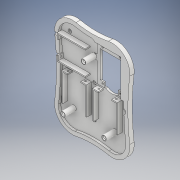
# Autodesk Inventor part: Chwytaka2_o
Saved by Autodesk Inventor 2017 (Build 210142000, 142)
## iProperties
Created: 2014-11-15
Part Number: Chwytaka2_o
Material: SolidWorks Materials|ABS
Document SubType Name: Modeling
Designer: Maciej
Density: 1.02 g/cm^3
Appearance: 255,255,255
Sending System: SolidWorks 2013
Last Author: Raymond Ma
Last Saved: 2015-02-18
Author: Maciej
Autodesk Inventor part; units mm, degrees
note: some values were not read from the file. Chosen so that the rebuilt part matches the saved one: arc direction of "Wyciągnięcie proste15".
ref_plane "YZ Plane" through (0, 0, 0) normal (1, 0, 0) x (0, 1, 0)
ref_plane "XZ Plane" through (0, 0, 0) normal (0, 1, 0) x (-1, 0, 0)
ref_plane "XY Plane" through (0, 0, 0) normal (0, 0, 1) x (1, 0, 0)
sketch "Szkic3" plane through (0, 0, 0) normal (0, 1, 0) x (-1, 0, 0)
  arc A0 (47.3256, 42.282) -> (47.3256, -32.282) centre (345, 5) ccw projected
  arc A1 (47.3256, -32.282) -> (47.3256, -32.282) centre (345, 5) ccw
  arc A2 (20.4082, -57.1046) -> (47.3256, -32.282) centre (25, -35.0782) ccw projected
  arc A3 (20.4082, -57.1046) -> (47.3256, -32.282) centre (25, -35.0782) ccw
  arc A4 (20.4082, -57.1046) -> (-20.4082, -57.1046) centre (0, -155) ccw projected
  arc A5 (20.4082, -57.1046) -> (-20.4082, -57.1046) centre (0, -155) ccw
  arc A6 (-47.3256, -32.282) -> (-20.4082, -57.1046) centre (-25, -35.0782) ccw projected
  arc A7 (-47.3256, -32.282) -> (-47.3256, -32.282) centre (-25, -35.0782) ccw
  arc A8 (-47.3256, -32.282) -> (-47.3256, 42.282) centre (-345, 5) ccw projected
  arc A9 (-47.3256, -32.282) -> (-47.3256, -32.282) centre (-345, 5) ccw
  arc A10 (-20.4082, 67.1046) -> (-47.3256, 42.282) centre (-25, 45.0782) ccw projected
  arc A11 (-20.4082, 67.1046) -> (-47.3256, 42.282) centre (-25, 45.0782) ccw
  arc A12 (-20.4082, 67.1046) -> (20.4082, 67.1046) centre (0, 165) ccw projected
  arc A13 (47.3256, 42.282) -> (20.4082, 67.1046) centre (25, 45.0782) ccw projected
  arc A14 (20.4082, 67.1046) -> (20.4082, 67.1046) centre (0, 165) ccw
  arc A15 (47.3256, 42.282) -> (20.4082, 67.1046) centre (25, 45.0782) ccw
  circle A16 centre (26, -30.3974) radius 1.5 projected
  circle A17 centre (26, -30.3974) radius 1.5
  circle A18 centre (26, -30.3974) radius 3
  circle A19 centre (-26, -30.3974) radius 1.5 projected
  circle A20 centre (-26, -30.3974) radius 1.5
  circle A21 centre (-26, -30.3974) radius 3
  circle A22 centre (-39, 0) radius 2.1526 projected
  circle A23 centre (-39, 0) radius 2.1526
  circle A24 centre (0, 10) radius 2.1526 projected
  circle A25 centre (0, 10) radius 2.1526
  circle A26 centre (31.0104, 51.0886) radius 2.1526 projected
  circle A27 centre (31.0104, 51.0886) radius 2.1526
  circle A28 centre (0, -30.3974) radius 2.1526
  circle A29 centre (0, 40) radius 1.5 projected
  circle A30 centre (0, 40) radius 1.5
  circle A31 centre (0, 40) radius 3
  arc A32 (-27.8847, 10.4357) -> (-15.5153, 10.4357) centre (-21.7, 22.4357) ccw projected
  circle A33 centre (-21.7, 22.4357) radius 13.5
  arc A34 (0, 60) -> (-3.7, 55.3715) centre (1.296, 55.1709) ccw
  arc A35 (-5.5975, 60.1493) -> (21.4286, 62.2098) centre (0, 165) ccw projected
  arc A36 (0, 60) -> (2.4776, 60.0292) centre (0, 165) ccw
  arc A37 (2.4776, 60.0292) -> (21.4286, 62.2098) centre (0, 165) ccw
  arc A38 (42.3644, 42.9034) -> (21.4286, 62.2098) centre (25, 45.0782) ccw projected
  arc A39 (42.3644, 42.9034) -> (40.5404, 23.1486) centre (345, 5) ccw
  arc A40 (21.4286, -52.2098) -> (42.3644, -32.9034) centre (25, -35.0782) ccw projected
  arc A41 (-42.3644, -32.9034) -> (-21.4286, -52.2098) centre (-25, -35.0782) ccw projected
  arc A42 (-42.3644, -32.9034) -> (-40.1293, -3.8798) centre (-345, 5) ccw projected
  arc A43 (-42.3644, -32.9034) -> (-21.4286, -52.2098) centre (-25, -35.0782) ccw
  arc A44 (-42.3644, -32.9034) -> (-40.1293, -3.8798) centre (-345, 5) ccw
  arc A45 (-40.1293, -3.8798) -> (-40.645, -2.9755) centre (-41.1289, -3.8507) ccw projected
  arc A46 (-40.5469, 3.0277) -> (-40.645, -2.9755) centre (-39, 0) ccw projected
  arc A47 (-40.645, -2.9755) -> (-40.645, -2.9755) centre (-39, 0) ccw
  arc A48 (-40.5469, 3.0277) -> (-40.0019, 3.9146) centre (-41.0019, 3.9182) ccw projected
  arc A49 (21.4286, -52.2098) -> (-21.4286, -52.2098) centre (0, -155) ccw
  line L0 (-7.45, 51.4857) -> (-7.45, 17.3857)
  line L1 (-7.45, 11.1857) -> (-35.95, 11.1857)
  line L2 (-3.7, 55.3715) -> (-3.7, 44) projected
  line L3 (-3.7, 55.3715) -> (-3.7, 44)
  arc A50 (-3.7, 44) -> (-2.7, 43) centre (-2.7, 44) ccw projected
  arc A51 (-3.7, 44) -> (-2.7, 43) centre (-2.7, 44) ccw
  line L4 (-2.7, 43) -> (0.0042, 43)
  circle A52 centre (0, 40) radius 3 projected
  arc A53 (-2.7, 37) -> (-3.7, 36) centre (-2.7, 36) ccw projected
  line L5 (0, 37) -> (-2.7, 37)
  line L6 (-3.7, 36) -> (-3.7, 14.2607) projected
  arc A54 (-2.7, 37) -> (-3.7, 36) centre (-2.7, 36) ccw
  line L7 (-3.7, 36) -> (-3.7, 11.1857)
  line L8 (-3.7, 11.1857) -> (-14.2376, 11.1857)
  line L9 (-40.0019, 3.9146) -> (-40.0019, 11.1857)
  line L10 (-40.0019, 11.1857) -> (-29.1624, 11.1857)
  line L11 (-7.45, 51.4857) -> (-35.95, 51.4857)
  circle A55 centre (-10.7, 54.4357) radius 1
  circle A56 centre (-32.7, 54.4357) radius 1
  line L12 (-7.45, 11.1857) -> (-10.7, 11.1857)
  circle A57 centre (-10.7, 14.6853) radius 1
  circle A58 centre (-32.7, 14.6853) radius 1
  line L13 (-7.45, 17.3857) -> (-12.95, 17.3857)
  line L14 (-12.95, 17.3857) -> (-12.95, 11.1857)
  line L15 (-7.45, 17.3857) -> (-7.45, 11.1857)
  line L16 (-35.95, 17.3857) -> (-35.95, 11.1857)
  line L17 (-7.45, 51.4857) -> (-7.45, 57.6857)
  line L18 (-7.45, 57.6857) -> (-13.65, 57.6857)
  line L19 (-13.65, 57.6857) -> (-13.65, 51.4857)
  line L20 (-35.95, 51.4857) -> (-35.95, 57.6857)
  line L21 (-35.95, 57.6857) -> (-29.75, 57.6857)
  line L22 (-29.75, 57.6857) -> (-29.75, 51.4857)
  line L23 (-3.741, 9.05) -> (-10.941, 9.05)
  line L24 (-10.941, 9.05) -> (-10.941, 7.55)
  line L25 (-10.941, 7.55) -> (-5.241, 7.55)
  line L26 (-5.241, 7.55) -> (-5.241, -26.45)
  line L27 (-5.241, -26.45) -> (-3.741, -26.45)
  line L28 (-3.741, -26.45) -> (-3.741, 9.05)
  line L29 (-35.241, 9.05) -> (-28.041, 9.05)
  line L30 (-28.041, 9.05) -> (-28.041, 7.55)
  line L31 (-28.041, 7.55) -> (-33.741, 7.55)
  line L32 (-33.741, 7.55) -> (-33.741, -26.45)
  line L33 (-35.241, -26.45) -> (-35.241, 9.05)
  line L34 (-33.741, -26.45) -> (-35.241, -26.45)
  line L35 (3.741, 9.05) -> (10.941, 9.05)
  line L36 (10.941, 9.05) -> (10.941, 7.55)
  line L37 (10.941, 7.55) -> (5.241, 7.55)
  line L38 (5.241, 7.55) -> (5.241, -26.45)
  line L39 (5.241, -26.45) -> (3.741, -26.45)
  line L40 (3.741, -26.45) -> (3.741, 9.05)
  line L41 (33.741, 7.55) -> (33.741, -26.45)
  line L42 (35.241, -26.45) -> (35.241, 9.05)
  line L43 (28.041, 9.05) -> (28.041, 7.55)
  line L44 (35.241, 9.05) -> (28.041, 9.05)
  line L45 (28.041, 7.55) -> (33.741, 7.55)
  line L46 (33.741, -26.45) -> (35.241, -26.45)
  line L47 (41.0774, 47.4486) -> (41.0774, 40.2486)
  line L48 (41.0774, 40.2486) -> (39.5774, 40.2486)
  line L49 (39.5774, 40.2486) -> (39.5774, 45.9486)
  line L50 (39.5774, 45.9486) -> (5.5774, 45.9486)
  line L51 (5.5774, 45.9486) -> (5.5774, 47.4486)
  line L52 (5.5774, 47.4486) -> (41.0774, 47.4486)
  line L53 (41.0774, 15.9486) -> (41.0774, 23.1486)
  line L54 (41.0774, 23.1486) -> (39.5774, 23.1486)
  line L55 (39.5774, 23.1486) -> (39.5774, 17.4486)
  line L56 (39.5774, 17.4486) -> (5.5774, 17.4486)
  line L57 (5.5774, 17.4486) -> (5.5774, 15.9486)
  line L58 (5.5774, 15.9486) -> (40.1966, 15.9486)
  arc A59 (40.1966, 15.9486) -> (42.3644, -32.9034) centre (345, 5) ccw
  line L59 (40.1966, 15.9486) -> (41.0774, 15.9486)
  circle A60 centre (-18.5, -1.35) radius 5 projected
  circle A61 centre (-18.5, -1.35) radius 5
  circle A62 centre (3.8019, -10.2171) radius 5 projected
  circle A63 centre (3.8019, -10.2171) radius 5
  line L60 (-35.95, 11.1857) -> (-30.45, 11.1857)
  line L61 (-35.95, 17.3857) -> (-35.95, 11.1857)
  line L62 (-12.95, 11.1857) -> (-7.45, 11.1857)
  line L63 (-7.45, 11.1857) -> (-7.45, 17.3857)
  line L64 (-7.45, 17.3857) -> (-12.95, 17.3857)
  line L65 (-12.95, 17.3857) -> (-12.95, 11.1857)
  line L66 (5.5774, 15.9486) -> (41.0774, 15.9486)
  line L67 (41.0774, 15.9486) -> (41.0774, 17.4486)
  line L68 (41.0774, 17.4486) -> (5.5774, 17.4486)
  line L69 (5.5774, 17.4486) -> (5.5774, 15.9486)
  line L70 (41.0774, 23.1486) -> (39.5774, 23.1486)
  line L71 (39.5774, 23.1486) -> (39.5774, 17.4486)
  line L72 (39.5774, 17.4486) -> (41.0774, 17.4486)
  line L73 (41.0774, 17.4486) -> (41.0774, 23.1486)
  line L74 (5.5774, 45.9486) -> (41.0774, 45.9486)
  line L75 (41.0774, 45.9486) -> (41.0774, 47.4486)
  line L76 (41.0774, 47.4486) -> (5.5774, 47.4486)
  line L77 (5.5774, 47.4486) -> (5.5774, 45.9486)
  line L78 (41.0774, 40.2486) -> (39.5774, 40.2486)
  line L79 (39.5774, 40.2486) -> (39.5774, 45.9486)
  line L80 (39.5774, 45.9486) -> (41.0774, 45.9486)
  line L81 (41.0774, 45.9486) -> (41.0774, 40.2486)
  line L82 (3.741, -26.45) -> (5.241, -26.45)
  line L83 (5.241, -26.45) -> (5.241, 9.05)
  line L84 (5.241, 9.05) -> (3.741, 9.05)
  line L85 (3.741, 9.05) -> (3.741, -26.45)
  line L86 (10.941, 9.05) -> (5.241, 9.05)
  line L87 (5.241, 9.05) -> (5.241, 7.55)
  line L88 (5.241, 7.55) -> (10.941, 7.55)
  line L89 (10.941, 7.55) -> (10.941, 9.05)
  line L90 (33.741, -26.45) -> (35.241, -26.45)
  line L91 (35.241, -26.45) -> (35.241, 9.05)
  line L92 (35.241, 9.05) -> (33.741, 9.05)
  line L93 (33.741, 9.05) -> (33.741, -26.45)
  line L94 (28.041, 7.55) -> (33.741, 7.55)
  line L95 (33.741, 7.55) -> (33.741, 9.05)
  line L96 (33.741, 9.05) -> (28.041, 9.05)
  line L97 (28.041, 9.05) -> (28.041, 7.55)
  line L98 (-35.241, -26.45) -> (-33.741, -26.45)
  line L99 (-33.741, -26.45) -> (-33.741, 9.05)
  line L100 (-33.741, 9.05) -> (-35.241, 9.05)
  line L101 (-35.241, 9.05) -> (-35.241, -26.45)
  line L102 (-33.741, 9.05) -> (-28.041, 9.05)
  line L103 (-28.041, 9.05) -> (-28.041, 7.55)
  line L104 (-28.041, 7.55) -> (-33.741, 7.55)
  line L105 (-33.741, 7.55) -> (-33.741, 9.05)
  line L106 (-10.941, 7.55) -> (-3.741, 7.55)
  line L107 (-3.741, 7.55) -> (-3.741, 9.05)
  line L108 (-3.741, 9.05) -> (-10.941, 9.05)
  line L109 (-10.941, 9.05) -> (-10.941, 7.55)
  line L110 (-3.741, 7.55) -> (-5.241, 7.55)
  line L111 (-5.241, 7.55) -> (-5.241, -26.45)
  line L112 (-5.241, -26.45) -> (-3.741, -26.45)
  line L113 (-3.741, -26.45) -> (-3.741, 7.55)
  line L114 (-13.65, 51.4857) -> (-7.45, 51.4857)
  line L115 (-7.45, 51.4857) -> (-7.45, 57.6857)
  line L116 (-7.45, 57.6857) -> (-13.65, 57.6857)
  line L117 (-13.65, 57.6857) -> (-13.65, 51.4857)
  line L118 (-35.95, 51.4857) -> (-29.75, 51.4857)
  line L119 (-29.75, 51.4857) -> (-29.75, 57.6857)
  line L120 (-29.75, 57.6857) -> (-35.95, 57.6857)
  line L121 (-35.95, 57.6857) -> (-35.95, 51.4857)
  line L122 (-35.95, 51.4857) -> (-7.45, 51.4857)
  line L123 (-7.45, 51.4857) -> (-7.45, 11.1857)
  line L124 (-7.45, 11.1857) -> (-35.95, 11.1857)
  line L125 (-35.95, 11.1857) -> (-35.95, 51.4857)
  line L126 (-35.95, 11.1857) -> (-30.45, 11.1857)
  line L127 (-30.45, 11.1857) -> (-30.45, 17.3857)
  line L128 (-30.45, 17.3857) -> (-35.95, 17.3857)
  line L129 (-35.95, 17.3857) -> (-35.95, 11.1857)
  line L130 (-29.75, 57.6857) -> (-13.65, 57.6857)
  line L131 (-13.65, 57.6857) -> (-13.65, 51.4857)
  line L132 (-13.65, 51.4857) -> (-29.75, 51.4857)
  line L133 (-29.75, 51.4857) -> (-29.75, 57.6857)
  line L134 (-7.45, 57.6857) -> (-3.0256, 57.6857)
  point P0 (0, 0)
  point P1 (-3.9929, 56.0786)
  point P2 (25, 18.319)
  point P3 (25, 18.319)
  point P4 (25, 18.319)
  dimension "d0" = 5
  dimension "d1" = 105
  dimension "d12" = 2
  dimension "d15" = 2
  dimension "d18" = 2
  dimension "d24" = 5.5
  dimension "d26" = 6.2
  dimension "d27" = 6.2
  dimension "d28" = 6.2
  dimension "d29" = 6.2
  dimension "d32" = 7.2
  dimension "d33" = 1.5
  dimension "d34" = 5.7
  dimension "d35" = 34
  dimension "d36" = 1.5
  dimension "d40" = 7.2
  dimension "d41" = 1.5
  dimension "d42" = 5.7
  dimension "d45" = 5.5
  constraints: 266 end point, 37 equal length, 37 point on circle, 36 perpendicular, 31 centre point, 22 horizontal, 14 point on line, 12 coincident, 5 vertical, 3 tangent, 2 concentric, 20 other
  measures "d0" radius of A34
  measures "d1" radius of A49
  measures "d12" diameter of A55
  measures "d15" diameter of A56
  measures "d18" diameter of A57
  measures "d24" distance of L0.end L13.end
  measures "d26" distance of L0.start L17.end
  measures "d27" distance of L17.end L18.end
  measures "d28" distance of L11.end L20.end
  measures "d29" distance of L20.end L21.end
  measures "d32" distance of L23.start L23.end
  measures "d33" distance of L23.end L24.end
  measures "d34" distance of L24.end L25.end
  measures "d35" distance of L25.end L26.end
  measures "d36" distance of L26.end L27.end
  measures "d40" distance of L47.start L47.end
  measures "d41" distance of L47.end L48.end
  measures "d42" distance of L48.end L49.end
  measures "d45" distance of L128.end L127.end
extrude "Wyciągnięcie proste14" add sketch "Szkic3" along normal blind 1.5 contours A49 A41 A42 A7 L33 L34 L32 L26 L27 | A7 L27 L28 L23 L24 L25 L26 L32 L31 L30 L29 L33 A42 A45 A47 A48 L9 L10 L1 A33 A32 L8 L7 L6 A53 L5 A31 L4 A50 L2 A34 A35 A38 A39 L54 L55 L56 L57 L58 A59 A40 A49 | A46 A47
extrude "Wyciągnięcie proste15" add sketch "Szkic3" along normal blind 1.5 contours A0 A2 A4 A7 A49 A40 A59 L59 L53 L54 A39 A38 A35 A34 L134 L18 L130 L21 L20 L125 L16 L10 L9 A48 A46 A45 A42 A8 A10 A12 A13 | A6 A7 A42 A41 A49 | L17 L134 A34 L2 A50 L4 A31 L5 A53 L6 L7 L8 L15 L0
extrude "Wyciągnięcie proste16" add sketch "Szkic3" along normal blind 1.5 contours A31
extrude "Wyciągnięcie proste17" add sketch "Szkic3" along normal blind 1.5 contours L58 L57 L56 L68 L53 L59 | L68 L55 L54 L53 | L47 L74 L50 L51 L52 | L47 L48 L49 L74
extrude "Wyciągnięcie proste18" add sketch "Szkic3" along normal blind 1.5 contours L35 L83 L38 A62 L40 | L35 L36 L37 L83 | A62 L38 L40 | A62 L38 L39 L40 | L93 L44 L42 L46 L41 | L45 L43 L44 L93
extrude "Wyciągnięcie proste19" add sketch "Szkic3" along normal blind 1.5 contours L33 L29 L99 L32 A7 | A7 L32 L34 L33 | L99 L29 L30 L31 | L25 L24 L23 L28 L106
extrude "Wyciągnięcie proste20" add sketch "Szkic3" along normal blind 1.5 contours L27 L26 A7 | A7 L26 L106 L28 L27 | L25 L24 L23 L28 L106
hole "Otwór4" at (-3.8019, 0, -10.2171) direction (0, 1, 0) diameter 10 depth 1.5
extrude "Wyciągnięcie proste21" add sketch "Szkic3" along normal blind 1.5 contours A21
extrude "Wyciągnięcie proste22" add sketch "Szkic3" along normal blind 1.5 contours A18
extrude "Wyciągnięcie proste24" add sketch "Szkic3" against normal blind 1.5 contours L16 L128 A33 A58 L127 L1 | A33 A58 L128 L127 | L20 L21 L22 L11 | L22 L130 L19 L11 | L14 L13 A33 A57 | A33 A57 L13 L15 L1 L14 | L19 L18 L17 L11
extrude "Wyciągnięcie proste25" add sketch "Szkic3" against normal blind 7.2 contours L58 L57 L56 L68 L53 L59 | L68 L55 L54 L53 | L47 L74 L50 L51 L52 | L47 L48 L49 L74
extrude "Wyciągnięcie proste26" add sketch "Szkic3" against normal blind 7.2 contours L35 L83 L38 A62 L40 | L35 L36 L37 L83 | A62 L38 L40 | A62 L38 L39 L40 | L93 L44 L42 L46 L41 | L45 L43 L44 L93
extrude "Wyciągnięcie proste27" add sketch "Szkic3" against normal blind 7.2 contours L33 L29 L99 L32 A7 | A7 L32 L34 L33 | L27 L26 A7 | A7 L26 L106 L28 L27 | L99 L29 L30 L31 | L25 L24 L23 L28 L106
extrude "Wyciągnięcie proste28" add sketch "Szkic3" against normal blind 4 contours A0 A2 A4 A7 A49 A40 A59 L59 L53 L54 A39 A38 A35 A34 L134 L18 L130 L21 L20 L125 L16 L10 L9 A48 A46 A45 A42 A8 A10 A12 A13 | A6 A7 A42 A41 A49
extrude "Wyciągnięcie proste29" add sketch "Szkic3" against normal blind 1.5 contours L17 L134 A34 L2 A50 L4 A31 L5 A53 L6 L7 L8 L15 L0
extrude "Wyciągnięcie proste30" add sketch "Szkic3" against normal blind 15 contours A18
extrude "Wyciągnięcie proste31" add sketch "Szkic3" against normal blind 15 contours A21
extrude "Wyciągnięcie proste32" add sketch "Szkic3" against normal blind 15 contours A31
fillet "Zaokrąglenie1" radius 1 1 edges at (1.5, -15, 40)
fillet "Zaokrąglenie2" radius 1 1 edges at (-24.5, -15, -30.3974)
fillet "Zaokrąglenie3" radius 1 1 edges at (27.5, -15, -30.3974)
extrude "Wyciągnięcie proste33" add sketch "Szkic3" against normal blind 1 contours A49 A41 A42 A7 L33 L34 L32 L26 L27 | A31 | A7 L27 L28 L23 L24 L25 L26 L32 L31 L30 L29 L33 A42 A45 A47 A48 L9 L10 L1 A33 A32 L8 L7 L6 A53 L5 A31 L4 A50 L2 A34 A35 A38 A39 L54 L55 L56 L57 L58 A59 A40 A49 | L33 L29 L99 L32 A7 | A7 L32 L34 L33 | L27 L26 A7 | A7 L26 L106 L28 L27 | A46 A47 | L99 L29 L30 L31 | L25 L24 L23 L28 L106 | A16 | A18 | A19 | A21 | A22 | A24 | A26 | A28 | A29 | L35 L83 L38 A62 L40 | L35 L36 L37 L83 | A62 L38 L40 | L40 A62 | A62 L38 L39 L40 | A62 L38 | L93 L44 L42 L46 L41 | L45 L43 L44 L93 | L47 L74 L50 L51 L52 | L47 L48 L49 L74 | A60
hole "Otwór5" at (39, 0, 0) direction (0, -1, 0) diameter 4.305 depth 1.5
hole "Otwór6" at (0, 0, 10) direction (0, -1, 0) diameter 4.305 depth 1.5
hole "Otwór7" at (0, 0, -30.3974) at (-31.0104, 0, 51.0886) direction (0, -1, 0) diameter 4.305 depth 1.5
hole "Otwór8" at (0, 0, 40) direction (0, -1, 0) diameter 3 depth 1.5
hole "Otwór9" at (-26, 0, -30.3974) at (26, 0, -30.3974) direction (0, -1, 0) diameter 3 depth 1.5
sketch "Szkic4" plane through (-39.5774, -7.2, 23.1486) normal (1, 0, 0) x (0, 0, -1)
  point P0 (23.1486, 7.2)
sketch "Szkic5" plane through (-39.5774, -7.2, 23.1486) normal (1, 0, 0) x (0, 0, -1)
  circle A0 centre (2.4873, 3.2928) radius 1
  circle A1 centre (2.4873, 3.2928) radius 1.5
  point P0 (23.1486, 7.2)
  dimension "d182" = 2
  dimension "d244" = 3
  constraints: 2 centre point, 1 coincident
  measures "d182" diameter of A0
  measures "d244" diameter of A1
sketch "Szkic6" plane through (-39.5774, -7.2, 45.9486) normal (1, 0, 0) x (0, 0, -1)
  point P0 (45.9486, 7.2)
sketch "Szkic7" plane through (-39.5774, -7.2, 45.9486) normal (1, 0, 0) x (0, 0, -1)
  line L0 (5.7, 0) -> (0, 0) projected
  circle A0 centre (3.25, 3.25) radius 1
  circle A1 centre (3.25, 3.25) radius 1.5
  point P0 (45.9486, 7.2)
  dimension "d185" = 2
  dimension "d241" = 3
  constraints: 2 centre point, 1 coincident
  measures "d185" diameter of A0
  measures "d241" diameter of A1
sketch "Szkic8" plane through (-28.041, -7.2, 7.55) normal (0, 0, -1) x (-1, 0, 0)
  line L0 (5.7, 6.2) -> (5.7, 0) projected
  circle A0 centre (2.45, 3.25) radius 1
  point P0 (-28.041, 7.2)
  dimension "d188" = 2
  constraints: 1 centre point
  measures "d188" diameter of A0
sketch "Szkic9" plane through (-5.241, -7.2, 7.55) normal (0, 0, -1) x (-1, 0, 0)
  circle A0 centre (3.2836, 3.3322) radius 1
  point P0 (-5.241, 7.2)
  dimension "d191" = 2
  constraints: 1 centre point
  measures "d191" diameter of A0
sketch "Szkic10" plane through (10.941, -7.2, 7.55) normal (0, 0, -1) x (-1, 0, 0)
  line L0 (0, 6.2) -> (0, 0) projected
  circle A0 centre (2.45, 3.25) radius 1
  point P0 (10.941, 7.2)
  dimension "d194" = 2
  constraints: 1 centre point
  measures "d194" diameter of A0
sketch "Szkic11" plane through (33.741, -7.2, 7.55) normal (0, 0, -1) x (-1, 0, 0)
  line L0 (5.7, 6.2) -> (5.7, 0) projected
  circle A0 centre (3.25, 3.25) radius 1
  point P0 (33.741, 7.2)
  dimension "d198" = 2
  constraints: 1 centre point
  measures "d198" diameter of A0
hole "Otwór10" at (8.491, -3.95, 7.55) direction (0, 0, 1) diameter 2 depth 1.5
hole "Otwór11" at (30.491, -3.95, 7.55) direction (0, 0, 1) diameter 2 depth 1.5
hole "Otwór12" at (-8.5246, -3.8678, 7.55) direction (0, 0, 1) diameter 2 depth 1.5
hole "Otwór13" at (-30.491, -3.95, 7.55) direction (0, 0, 1) diameter 2 depth 1.5
hole "Otwór14" at (-39.5774, -3.95, 42.6986) direction (-1, 0, 0) diameter 3 depth 10
hole "Otwór15" at (-39.5774, -3.9072, 20.6612) direction (-1, 0, 0) diameter 3 depth 10
extrude "Wyciągnięcie proste34" add sketch "Szkic7" against normal blind 1.5
extrude "Wyciągnięcie proste35" add sketch "Szkic5" against normal blind 1.5
hole "Otwór16" at (32.7, 0, 14.6853) direction (0, -1, 0) diameter 2 depth 1.5 counterbore diameter 3 counterbore depth 0.75
hole "Otwór17" at (10.7, 0, 14.6853) direction (0, -1, 0) diameter 2 depth 1.5 counterbore diameter 3 counterbore depth 0.75
hole "Otwór18" at (10.7, 0, 54.4357) direction (0, -1, 0) diameter 2 depth 1.5 counterbore diameter 3 counterbore depth 0.75
hole "Otwór19" at (32.7, 0, 54.4357) direction (0, -1, 0) diameter 2 depth 1.5 counterbore diameter 3 counterbore depth 0.75
